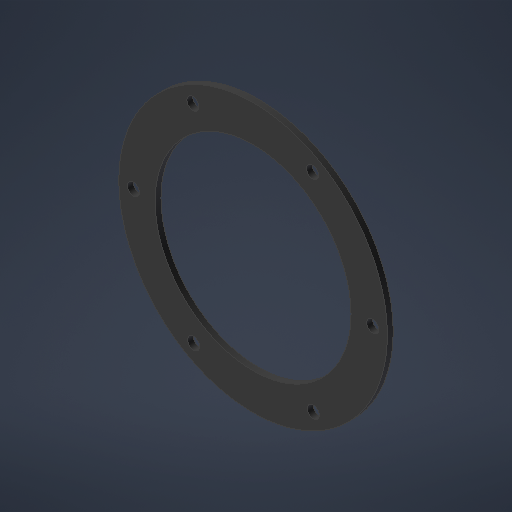
# Autodesk Inventor part: stator_mount_ret
Saved by Autodesk Inventor 2026.1 (Build 301233000, 233)
## iProperties
Created: 2026-04-16
Part Number: stator_mount_ret
Material: Generic
Document SubType Name: Modeling
Designer: aaron
Density: 1 g/cm^3
Appearance: Default
Author: aaron
Autodesk Inventor part; units mm, degrees
ref_plane "YZ Plane" through (0, 0, 0) normal (1, 0, 0) x (0, 1, 0)
ref_plane "XZ Plane" through (0, 0, 0) normal (0, 1, 0) x (-1, 0, 0)
ref_plane "XY Plane" through (0, 0, 0) normal (0, 0, 1) x (1, 0, 0)
sketch "Sketch1" plane through (0, 0, 0) normal (0, 0, 1) x (1, 0, 0)
  circle A0 centre (0, 0) radius 29
  circle A1 centre (0, 0) radius 27
  circle A2 centre (0, 0) radius 37
  dimension "d0" = 58
  dimension "d1" = 2
  dimension "d2" = 8
  constraints: 3 centre point, 1 coincident
  measures "d0" diameter of A0
  measures "d1" radial gap between concentric circles of A0 A1
  measures "d2" radial gap between concentric circles of A0 A2
extrude "Extrusion1" add sketch "Sketch1" along normal blind 1.6 contours A0 | A2
sketch "Sketch2" plane through (0, 0, 1.6) normal (0, 0, 1) x (1, 0, 0)
  circle A0 centre (-32.9998, -0.1189) radius 1.25 projected
  circle A1 centre (-16.3969, -28.6381) radius 1.25 projected
  circle A2 centre (-16.6029, 28.5192) radius 1.25 projected
  circle A3 centre (16.3969, 28.6381) radius 1.25 projected
  circle A4 centre (16.6029, -28.5192) radius 1.25 projected
  circle A5 centre (32.9998, 0.1189) radius 1.25 projected
  circle A6 centre (-32.9998, -0.1189) radius 1.65
  circle A7 centre (-16.3969, -28.6381) radius 1.65
  circle A8 centre (16.6029, -28.5192) radius 1.65
  circle A9 centre (32.9998, 0.1189) radius 1.65
  circle A10 centre (16.3969, 28.6381) radius 1.65
  circle A11 centre (-16.6029, 28.5192) radius 1.65
  point P0 (0, 0)
  dimension "d5" = 3.3
  dimension "d8" = 360
  constraints: 6 centre point, 1 coincident, 13 other
  measures "d5" diameter of A6
extrude "Extrusion2" cut sketch "Sketch2" against normal through all contours A0 | A1 | A2 | A3 | A4 | A5 | A6 | A7 | A8 | A9 | A10 | A11
body "Solid1"
